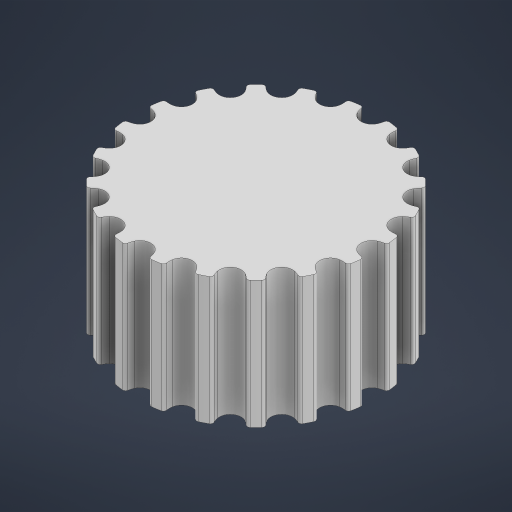
# Autodesk Inventor part: 2mm_GT2_Pully
Saved by Autodesk Inventor 2024.2 (Build 282272000, 272)
## iProperties
Created: 2026-01-11
Part Number: 2mm_GT2_Pully
Material: Generic
Document SubType Name: Modeling
Designer: 4aida
Density: 1 g/cm^3
Appearance: Default
Author: 4aida
Autodesk Inventor part; units mm, degrees
ref_plane "YZ Plane" through (0, 0, 0) normal (1, 0, 0) x (0, 1, 0)
ref_plane "XZ Plane" through (0, 0, 0) normal (0, 1, 0) x (-1, 0, 0)
ref_plane "XY Plane" through (0, 0, 0) normal (0, 0, 1) x (1, 0, 0)
sketch "Sketch1" plane through (0, 0, 0) normal (0, 1, 0) x (-1, 0, 0)
  circle A0 centre (0, 0) radius 6.7422 construction
  circle A1 centre (0, 0) radius 5.3622 construction
  circle A2 centre (0, 0) radius 6.1122 construction
  arc A3 (5.3622, 0) -> (5.674, -0.4989) centre (5.9172, 0) ccw
  arc A4 (6.0658, -0.7517) -> (5.9424, -0.5855) centre (5.9169, -0.7333) ccw
  arc A5 (5.674, -0.4989) -> (5.9424, -0.5855) centre (6.1122, 0.4) ccw
  circle A6 centre (0, 0) radius 6.3662 construction
  line L0 (0, 0) -> (6.0369, -0.9562) construction
  line L1 (5.9172, 0) -> (0, 0) construction
  arc A7 (5.5505, -1.2789) -> (5.0998, -1.657) centre (5.6276, -1.8285) ccw
  arc A8 (5.8325, -1.2795) -> (6.0012, -1.1595) centre (5.8539, -1.131) ccw
  arc A9 (5.8325, -1.2795) -> (5.5505, -1.2789) centre (5.6894, -2.2692) ccw
  arc A10 (6.0012, -1.1595) -> (6.0658, -0.7517) centre (0, 0) ccw
  arc A11 (5.9424, 0.5855) -> (5.674, 0.4989) centre (6.1122, -0.4) ccw
  arc A12 (5.674, 0.4989) -> (5.3622, 0) centre (5.9172, 0) ccw
  arc A13 (5.9424, 0.5855) -> (6.0658, 0.7517) centre (5.9169, 0.7333) ccw
  arc A14 (6.0658, 0.7517) -> (6.0012, 1.1595) centre (0, 0) ccw
  arc A15 (6.0012, 1.1595) -> (5.8325, 1.2795) centre (5.8539, 1.131) ccw
  arc A16 (5.5505, 1.2789) -> (5.8325, 1.2795) centre (5.6894, 2.2692) ccw
  arc A17 (5.0998, 1.657) -> (5.5505, 1.2789) centre (5.6276, 1.8285) ccw
  arc A18 (5.4706, 2.3931) -> (5.2421, 2.2278) centre (5.9367, 1.5084) ccw
  arc A19 (5.2421, 2.2278) -> (5.0998, 1.657) centre (5.6276, 1.8285) ccw
  arc A20 (5.4706, 2.3931) -> (5.5366, 2.5894) centre (5.4007, 2.5258) ccw
  arc A21 (5.5366, 2.5894) -> (5.3492, 2.9572) centre (0, 0) ccw
  arc A22 (5.3492, 2.9572) -> (5.1516, 3.0192) centre (5.2179, 2.8846) ccw
  arc A23 (4.8836, 2.9315) -> (5.1516, 3.0192) centre (4.7098, 3.9163) ccw
  arc A24 (4.3381, 3.1518) -> (4.8836, 2.9315) centre (4.7871, 3.478) ccw
  arc A25 (4.4634, 3.9665) -> (4.2971, 3.7387) centre (5.18, 3.2691) ccw
  arc A26 (4.2971, 3.7387) -> (4.3381, 3.1518) centre (4.7871, 3.478) ccw
  arc A27 (4.4634, 3.9665) -> (4.4655, 4.1736) centre (4.3559, 4.0711) ccw
  arc A28 (4.4655, 4.1736) -> (4.1736, 4.4655) centre (0, 0) ccw
  arc A29 (4.1736, 4.4655) -> (3.9665, 4.4634) centre (4.0711, 4.3559) ccw
  arc A30 (3.7387, 4.2971) -> (3.9665, 4.4634) centre (3.2691, 5.18) ccw
  arc A31 (3.1518, 4.3381) -> (3.7387, 4.2971) centre (3.478, 4.7871) ccw
  arc A32 (3.0192, 5.1516) -> (2.9315, 4.8836) centre (3.9163, 4.7098) ccw
  arc A33 (2.9315, 4.8836) -> (3.1518, 4.3381) centre (3.478, 4.7871) ccw
  arc A34 (3.0192, 5.1516) -> (2.9572, 5.3492) centre (2.8846, 5.2179) ccw
  arc A35 (2.9572, 5.3492) -> (2.5894, 5.5366) centre (0, 0) ccw
  arc A36 (2.5894, 5.5366) -> (2.3931, 5.4706) centre (2.5258, 5.4007) ccw
  arc A37 (2.2278, 5.2421) -> (2.3931, 5.4706) centre (1.5084, 5.9367) ccw
  arc A38 (1.657, 5.0998) -> (2.2278, 5.2421) centre (1.8285, 5.6276) ccw
  arc A39 (1.2795, 5.8325) -> (1.2789, 5.5505) centre (2.2692, 5.6894) ccw
  arc A40 (1.2789, 5.5505) -> (1.657, 5.0998) centre (1.8285, 5.6276) ccw
  arc A41 (1.2795, 5.8325) -> (1.1595, 6.0012) centre (1.131, 5.8539) ccw
  arc A42 (1.1595, 6.0012) -> (0.7517, 6.0658) centre (0, 0) ccw
  arc A43 (0.7517, 6.0658) -> (0.5855, 5.9424) centre (0.7333, 5.9169) ccw
  arc A44 (0.4989, 5.674) -> (0.5855, 5.9424) centre (-0.4, 6.1122) ccw
  arc A45 (0, 5.3622) -> (0.4989, 5.674) centre (0, 5.9172) ccw
  arc A46 (-0.5855, 5.9424) -> (-0.4989, 5.674) centre (0.4, 6.1122) ccw
  arc A47 (-0.4989, 5.674) -> (0, 5.3622) centre (0, 5.9172) ccw
  arc A48 (-0.5855, 5.9424) -> (-0.7517, 6.0658) centre (-0.7333, 5.9169) ccw
  arc A49 (-0.7517, 6.0658) -> (-1.1595, 6.0012) centre (0, 0) ccw
  arc A50 (-1.1595, 6.0012) -> (-1.2795, 5.8325) centre (-1.131, 5.8539) ccw
  arc A51 (-1.2789, 5.5505) -> (-1.2795, 5.8325) centre (-2.2692, 5.6894) ccw
  arc A52 (-1.657, 5.0998) -> (-1.2789, 5.5505) centre (-1.8285, 5.6276) ccw
  arc A53 (-2.3931, 5.4706) -> (-2.2278, 5.2421) centre (-1.5084, 5.9367) ccw
  arc A54 (-2.2278, 5.2421) -> (-1.657, 5.0998) centre (-1.8285, 5.6276) ccw
  arc A55 (-2.3931, 5.4706) -> (-2.5894, 5.5366) centre (-2.5258, 5.4007) ccw
  arc A56 (-2.5894, 5.5366) -> (-2.9572, 5.3492) centre (0, 0) ccw
  arc A57 (-2.9572, 5.3492) -> (-3.0192, 5.1516) centre (-2.8846, 5.2179) ccw
  arc A58 (-2.9315, 4.8836) -> (-3.0192, 5.1516) centre (-3.9163, 4.7098) ccw
  arc A59 (-3.1518, 4.3381) -> (-2.9315, 4.8836) centre (-3.478, 4.7871) ccw
  arc A60 (-3.9665, 4.4634) -> (-3.7387, 4.2971) centre (-3.2691, 5.18) ccw
  arc A61 (-3.7387, 4.2971) -> (-3.1518, 4.3381) centre (-3.478, 4.7871) ccw
  arc A62 (-3.9665, 4.4634) -> (-4.1736, 4.4655) centre (-4.0711, 4.3559) ccw
  arc A63 (-4.1736, 4.4655) -> (-4.4655, 4.1736) centre (0, 0) ccw
  arc A64 (-4.4655, 4.1736) -> (-4.4634, 3.9665) centre (-4.3559, 4.0711) ccw
  arc A65 (-4.2971, 3.7387) -> (-4.4634, 3.9665) centre (-5.18, 3.2691) ccw
  arc A66 (-4.3381, 3.1518) -> (-4.2971, 3.7387) centre (-4.7871, 3.478) ccw
  arc A67 (-5.1516, 3.0192) -> (-4.8836, 2.9315) centre (-4.7098, 3.9163) ccw
  arc A68 (-4.8836, 2.9315) -> (-4.3381, 3.1518) centre (-4.7871, 3.478) ccw
  arc A69 (-5.1516, 3.0192) -> (-5.3492, 2.9572) centre (-5.2179, 2.8846) ccw
  arc A70 (-5.3492, 2.9572) -> (-5.5366, 2.5894) centre (0, 0) ccw
  arc A71 (-5.5366, 2.5894) -> (-5.4706, 2.3931) centre (-5.4007, 2.5258) ccw
  arc A72 (-5.2421, 2.2278) -> (-5.4706, 2.3931) centre (-5.9367, 1.5084) ccw
  arc A73 (-5.0998, 1.657) -> (-5.2421, 2.2278) centre (-5.6276, 1.8285) ccw
  arc A74 (-5.8325, 1.2795) -> (-5.5505, 1.2789) centre (-5.6894, 2.2692) ccw
  arc A75 (-5.5505, 1.2789) -> (-5.0998, 1.657) centre (-5.6276, 1.8285) ccw
  arc A76 (-5.8325, 1.2795) -> (-6.0012, 1.1595) centre (-5.8539, 1.131) ccw
  arc A77 (-6.0012, 1.1595) -> (-6.0658, 0.7517) centre (0, 0) ccw
  arc A78 (-6.0658, 0.7517) -> (-5.9424, 0.5855) centre (-5.9169, 0.7333) ccw
  arc A79 (-5.674, 0.4989) -> (-5.9424, 0.5855) centre (-6.1122, -0.4) ccw
  arc A80 (-5.3622, 0) -> (-5.674, 0.4989) centre (-5.9172, 0) ccw
  arc A81 (-5.9424, -0.5855) -> (-5.674, -0.4989) centre (-6.1122, 0.4) ccw
  arc A82 (-5.674, -0.4989) -> (-5.3622, 0) centre (-5.9172, 0) ccw
  arc A83 (-5.9424, -0.5855) -> (-6.0658, -0.7517) centre (-5.9169, -0.7333) ccw
  arc A84 (-6.0658, -0.7517) -> (-6.0012, -1.1595) centre (0, 0) ccw
  arc A85 (-6.0012, -1.1595) -> (-5.8325, -1.2795) centre (-5.8539, -1.131) ccw
  arc A86 (-5.5505, -1.2789) -> (-5.8325, -1.2795) centre (-5.6894, -2.2692) ccw
  arc A87 (-5.0998, -1.657) -> (-5.5505, -1.2789) centre (-5.6276, -1.8285) ccw
  arc A88 (-5.4706, -2.3931) -> (-5.2421, -2.2278) centre (-5.9367, -1.5084) ccw
  arc A89 (-5.2421, -2.2278) -> (-5.0998, -1.657) centre (-5.6276, -1.8285) ccw
  arc A90 (-5.4706, -2.3931) -> (-5.5366, -2.5894) centre (-5.4007, -2.5258) ccw
  arc A91 (-5.5366, -2.5894) -> (-5.3492, -2.9572) centre (0, 0) ccw
  arc A92 (-5.3492, -2.9572) -> (-5.1516, -3.0192) centre (-5.2179, -2.8846) ccw
  arc A93 (-4.8836, -2.9315) -> (-5.1516, -3.0192) centre (-4.7098, -3.9163) ccw
  arc A94 (-4.3381, -3.1518) -> (-4.8836, -2.9315) centre (-4.7871, -3.478) ccw
  arc A95 (-4.4634, -3.9665) -> (-4.2971, -3.7387) centre (-5.18, -3.2691) ccw
  arc A96 (-4.2971, -3.7387) -> (-4.3381, -3.1518) centre (-4.7871, -3.478) ccw
  arc A97 (-4.4634, -3.9665) -> (-4.4655, -4.1736) centre (-4.3559, -4.0711) ccw
  arc A98 (-4.4655, -4.1736) -> (-4.1736, -4.4655) centre (0, 0) ccw
  arc A99 (-4.1736, -4.4655) -> (-3.9665, -4.4634) centre (-4.0711, -4.3559) ccw
  arc A100 (-3.7387, -4.2971) -> (-3.9665, -4.4634) centre (-3.2691, -5.18) ccw
  arc A101 (-3.1518, -4.3381) -> (-3.7387, -4.2971) centre (-3.478, -4.7871) ccw
  arc A102 (-3.0192, -5.1516) -> (-2.9315, -4.8836) centre (-3.9163, -4.7098) ccw
  arc A103 (-2.9315, -4.8836) -> (-3.1518, -4.3381) centre (-3.478, -4.7871) ccw
  arc A104 (-3.0192, -5.1516) -> (-2.9572, -5.3492) centre (-2.8846, -5.2179) ccw
  arc A105 (-2.9572, -5.3492) -> (-2.5894, -5.5366) centre (0, 0) ccw
  arc A106 (-2.5894, -5.5366) -> (-2.3931, -5.4706) centre (-2.5258, -5.4007) ccw
  arc A107 (-2.2278, -5.2421) -> (-2.3931, -5.4706) centre (-1.5084, -5.9367) ccw
  arc A108 (-1.657, -5.0998) -> (-2.2278, -5.2421) centre (-1.8285, -5.6276) ccw
  arc A109 (-1.2795, -5.8325) -> (-1.2789, -5.5505) centre (-2.2692, -5.6894) ccw
  arc A110 (-1.2789, -5.5505) -> (-1.657, -5.0998) centre (-1.8285, -5.6276) ccw
  arc A111 (-1.2795, -5.8325) -> (-1.1595, -6.0012) centre (-1.131, -5.8539) ccw
  arc A112 (-1.1595, -6.0012) -> (-0.7517, -6.0658) centre (0, 0) ccw
  arc A113 (-0.7517, -6.0658) -> (-0.5855, -5.9424) centre (-0.7333, -5.9169) ccw
  arc A114 (-0.4989, -5.674) -> (-0.5855, -5.9424) centre (0.4, -6.1122) ccw
  arc A115 (0, -5.3622) -> (-0.4989, -5.674) centre (0, -5.9172) ccw
  arc A116 (0.5855, -5.9424) -> (0.4989, -5.674) centre (-0.4, -6.1122) ccw
  arc A117 (0.4989, -5.674) -> (0, -5.3622) centre (0, -5.9172) ccw
  arc A118 (0.5855, -5.9424) -> (0.7517, -6.0658) centre (0.7333, -5.9169) ccw
  arc A119 (0.7517, -6.0658) -> (1.1595, -6.0012) centre (0, 0) ccw
  arc A120 (1.1595, -6.0012) -> (1.2795, -5.8325) centre (1.131, -5.8539) ccw
  arc A121 (1.2789, -5.5505) -> (1.2795, -5.8325) centre (2.2692, -5.6894) ccw
  arc A122 (1.657, -5.0998) -> (1.2789, -5.5505) centre (1.8285, -5.6276) ccw
  arc A123 (2.3931, -5.4706) -> (2.2278, -5.2421) centre (1.5084, -5.9367) ccw
  arc A124 (2.2278, -5.2421) -> (1.657, -5.0998) centre (1.8285, -5.6276) ccw
  arc A125 (2.3931, -5.4706) -> (2.5894, -5.5366) centre (2.5258, -5.4007) ccw
  arc A126 (2.5894, -5.5366) -> (2.9572, -5.3492) centre (0, 0) ccw
  arc A127 (2.9572, -5.3492) -> (3.0192, -5.1516) centre (2.8846, -5.2179) ccw
  arc A128 (2.9315, -4.8836) -> (3.0192, -5.1516) centre (3.9163, -4.7098) ccw
  arc A129 (3.1518, -4.3381) -> (2.9315, -4.8836) centre (3.478, -4.7871) ccw
  arc A130 (3.9665, -4.4634) -> (3.7387, -4.2971) centre (3.2691, -5.18) ccw
  arc A131 (3.7387, -4.2971) -> (3.1518, -4.3381) centre (3.478, -4.7871) ccw
  arc A132 (3.9665, -4.4634) -> (4.1736, -4.4655) centre (4.0711, -4.3559) ccw
  arc A133 (4.1736, -4.4655) -> (4.4655, -4.1736) centre (0, 0) ccw
  arc A134 (4.4655, -4.1736) -> (4.4634, -3.9665) centre (4.3559, -4.0711) ccw
  arc A135 (4.2971, -3.7387) -> (4.4634, -3.9665) centre (5.18, -3.2691) ccw
  arc A136 (4.3381, -3.1518) -> (4.2971, -3.7387) centre (4.7871, -3.478) ccw
  arc A137 (5.1516, -3.0192) -> (4.8836, -2.9315) centre (4.7098, -3.9163) ccw
  arc A138 (4.8836, -2.9315) -> (4.3381, -3.1518) centre (4.7871, -3.478) ccw
  arc A139 (5.1516, -3.0192) -> (5.3492, -2.9572) centre (5.2179, -2.8846) ccw
  arc A140 (5.3492, -2.9572) -> (5.5366, -2.5894) centre (0, 0) ccw
  arc A141 (5.5366, -2.5894) -> (5.4706, -2.3931) centre (5.4007, -2.5258) ccw
  arc A142 (5.2421, -2.2278) -> (5.4706, -2.3931) centre (5.9367, -1.5084) ccw
  arc A143 (5.0998, -1.657) -> (5.2421, -2.2278) centre (5.6276, -1.8285) ccw
  point P0 (6.0369, 0.9562)
  point P1 (5.446, 2.7749)
  point P2 (4.322, 4.322)
  point P3 (2.7749, 5.446)
  point P4 (0.9562, 6.0369)
  point P5 (-0.9562, 6.0369)
  point P6 (-2.7749, 5.446)
  point P7 (-4.322, 4.322)
  point P8 (-5.446, 2.7749)
  point P9 (-6.0369, 0.9562)
  point P10 (-6.0369, -0.9562)
  point P11 (-5.446, -2.7749)
  point P12 (-4.322, -4.322)
  point P13 (-2.7749, -5.446)
  point P14 (-0.9562, -6.0369)
  point P15 (0.9562, -6.0369)
  point P16 (2.7749, -5.446)
  point P17 (4.322, -4.322)
  point P18 (5.446, -2.7749)
  point P19 (-3.1518, 4.3381)
  point P20 (-4.3381, -3.1518)
  point P21 (5.0998, -1.657)
  dimension "d0" = 0.555
  dimension "d1" = 1
  dimension "d2" = 1.38
  dimension "d3" = 0.75
  dimension "d4" = 0.254
  dimension "d5" = 0.4
  dimension "d6" = 12.7324
  dimension "d7" = 0.15
  dimension "d8" = 9
  dimension "d11" = 360
  constraints: 302 point on circle, 143 centre point, 7 symmetric about line, 4 coincident, 4 end point, 3 tangent, 2 horizontal alignment, 1 horizontal, 467 other
  measures "d0" radius of A3
  measures "d1" radius of A5
  measures "d4" radial gap between concentric circles of A2 A6
  measures "d5" vertical distance of L1.start A5.centre
  measures "d6" diameter of A6
  measures "d7" radius of A4
  measures "d8" angle of L0 L1
extrude "Extrusion1" add sketch "Sketch1" along normal blind 6.5
equation "\"d6\" = 0.63662 * R_"
equation "\"R_\" = 20"
body "Solid1"
